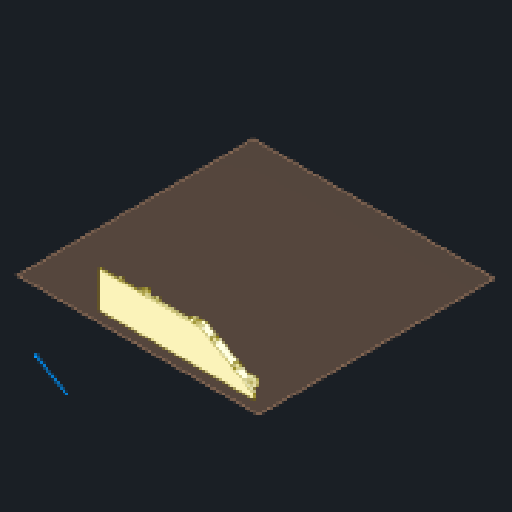
# Autodesk Inventor part: right_side
Saved by Autodesk Inventor 2023 (Build 270158000, 158)
## iProperties
Created: 2024-05-08
Part Number: right_side
Material: Nylon 6/6
Document SubType Name: Modeling
Designer: szymo
Density: 1.13 g/cm^3
Appearance: Nylon 6
Mass: 14.3001 g
Surface Area: 114.851 cm^2
Volume: 12.655 cm^3
Author: szymo
Autodesk Inventor part; units mm, degrees
ref_plane "YZ Plane" through (0, 0, 0) normal (1, 0, 0) x (0, 1, 0)
ref_plane "XZ Plane" through (0, 0, 0) normal (0, 1, 0) x (-1, 0, 0)
ref_plane "XY Plane" through (0, 0, 0) normal (0, 0, 1) x (1, 0, 0)
sketch "Sketch1" plane through (0, 0, 0) normal (0, 0, 1) x (1, 0, 0)
  line L0 (128, 8) -> (128, 3.5) projected
  line L1 (128, 3.5) -> (132, 3.5) projected
  line L2 (132, 3.5) -> (132, 0) projected
  line L3 (132, 0) -> (146, 0) projected
  line L4 (146, 0) -> (132, 9) projected
  line L5 (132, 9) -> (132, 8) projected
  line L6 (132, 8) -> (128, 8) projected
  circle A0 centre (-25, 12) radius 22.5 projected
  line L7 (116.5, 3.5) -> (116.5, 11.1395) projected
  line L8 (116.5, 14.6395) -> (116.5, 11.1395) projected
  line L9 (109.1155, 18.903) -> (116.5, 14.6395) projected
  line L10 (109.1155, 18.903) -> (83.8327, 33.5) projected
  line L11 (47.75, 33.5) -> (83.8327, 33.5) projected
  line L12 (0, 3.5) -> (0, 31) projected
  line L13 (0, 3.5) -> (0, 33.5)
  line L14 (0, 33.5) -> (83.8327, 33.5)
  line L15 (83.8327, 33.5) -> (128, 8)
  line L16 (128, 3.5) -> (0, 3.5)
  point P0 (0, 0)
  constraints: 8 end point, 2 collinear, 1 parallel, 1 point on line
extrude "Extrusion1" add sketch "Sketch1" against normal blind 2 contours L0 L16 L7 L8 L15 | L8 L7 L16 L12 L13 L14 L11 L10 L9
sketch "Sketch2" plane through (0, 0, -2) normal (0, 0, -1) x (-1, 0, 0)
  circle A0 centre (-15.375, 18.875) radius 13.7 projected
  line L0 (0, 33.5) -> (-83.8327, 33.5) projected
  line L1 (-128, 3.5) -> (0, 3.5) projected
  line L2 (-32.075, 33.5) -> (0, 33.5)
  line L3 (0, 33.5) -> (0, 3.5)
  line L4 (0, 3.5) -> (-32.075, 3.5)
  line L5 (-32.075, 3.5) -> (-32.075, 33.5)
  point P0 (0, 0)
  point P1 (-116.5, 3.5)
  dimension "d2" = 27.4
  dimension "d3" = 16.7
  constraints: 8 end point, 2 parallel, 1 horizontal, 1 perpendicular, 1 point on line
  measures "d2" diameter of A0
  measures "d3" distance from line of L5 A0.centre
extrude "Extrusion2" cut sketch "Sketch2" against normal blind 1 contours A0 | L3 L1 L5 L0
sketch "Sketch3" plane through (0, 0, -1) normal (0, 0, -1) x (-1, 0, 0)
  circle A0 centre (-15.375, 18.875) radius 13.7 projected
  line L0 (-32.075, 33.5) -> (0, 33.5) projected
  line L1 (-32.075, 3.5) -> (-32.075, 33.5) projected
  line L2 (0, 3.5) -> (-32.075, 3.5) projected
  line L3 (0, 33.5) -> (0, 3.5) projected
  line L4 (0, 3.5) -> (-128, 3.5) projected
  line L5 (0, 3.5) -> (-5, 3.5)
  line L6 (-5, 3.5) -> (-5, 6.5)
  line L7 (-5, 6.5) -> (0, 6.5)
  line L8 (0, 6.5) -> (0, 3.5)
  line L9 (-32.075, 3.5) -> (-27.075, 3.5)
  line L10 (-27.075, 3.5) -> (-27.075, 6.5)
  line L11 (-27.075, 6.5) -> (-32.075, 6.5)
  line L12 (-32.075, 6.5) -> (-32.075, 3.5)
  line L13 (-32.075, 9.5) -> (-25.365, 9.5)
  line L14 (-1.6801, 18.5) -> (0, 18.5)
  line L15 (0, 33.5) -> (0, 3.5) projected
  point P0 (0, 0)
  point P1 (-116.5, 3.5)
  point P2 (0, 18.5)
  dimension "d6" = 5
  dimension "d7" = 3
  dimension "d8" = 5
  dimension "d9" = 3
  dimension "d10" = 3
  constraints: 20 end point, 4 parallel, 3 perpendicular, 3 point on line, 2 horizontal, 2 point on circle, 1 midpoint
  measures "d6" distance of L6.end L7.end
  measures "d7" distance of L5.end L6.end
  measures "d8" distance of L11.end L10.end
  measures "d9" distance of L10.end L9.end
  measures "d10" distance between parallel lines of L13 L11
ref_plane "Work Plane1" through (1, 4.5, -18.6) normal (0, 0, 1) x (1, 0, 0)
ref_plane "Work Plane2" through (1.675, 5.175, -4.8) normal (0, 0, 1) x (1, 0, 0)
extrude "Extrusion3" add sketch "Sketch3" along normal blind 6.8 contours A0 L14 L3 L7 L6 L2 L10 L11 L1 L13 | L11 L10 L2 L1 | L3 L2 L6 L7
sketch "Sketch4" plane through (0, 0, -7.8) normal (0, 0, -1) x (-1, 0, 0)
  circle A0 centre (-15.375, 18.875) radius 13.7 projected
  line L0 (-1.6801, 18.5) -> (0, 18.5) projected
  line L1 (0, 33.5) -> (0, 18.5) projected
  line L2 (-32.075, 33.5) -> (0, 33.5) projected
  line L3 (-32.075, 9.5) -> (-32.075, 33.5) projected
  line L4 (-32.075, 9.5) -> (-25.365, 9.5) projected
  arc A1 (-25.365, 9.5) -> (-1.6801, 18.5) centre (-15.375, 18.875) ccw projected
  line L5 (-29.0741, 19.0336) -> (-32.075, 19.0336)
  line L6 (-32.075, 9.5) -> (-32.075, 33.5) projected
  line L7 (0, 18.5) -> (-1.6801, 18.5) projected
  line L8 (-1.6801, 18.5) -> (0, 18.5)
  arc A2 (-25.365, 9.5) -> (-1.6801, 18.5) centre (-15.375, 18.875) ccw projected
  line L9 (-25.365, 9.5) -> (-32.075, 9.5) projected
  line L10 (-32.075, 9.5) -> (-32.075, 3.5) projected
  line L11 (-32.075, 3.5) -> (0, 3.5) projected
  line L12 (0, 3.5) -> (0, 18.5) projected
  line L13 (0, 18.5) -> (-1.6801, 18.5) projected
  point P0 (0, 0)
  constraints: 4 end point, 1 collinear, 1 perpendicular, 1 point on line, 2 other
ref_plane "Work Plane3" through (1, 4.5, -18.6) normal (0, 0, 1) x (1, 0, 0)
extrude "Extrusion4" add sketch "Sketch4" along normal up to surface (10.8 mm away) contours A0 L4 L3 L5 | L0 L12 L11 L10 L4 A0
sketch "Sketch5" plane through (25.365, 9.5, -1) normal (0, 1, 0) x (1, 0, 0)
  line L0 (6.71, 0) -> (0, 0) projected
  line L1 (6.71, 1) -> (6.71, 0) projected
  line L2 (6.71, 1) -> (6.71, 6.8) projected
  line L3 (0, 6.8) -> (6.71, 6.8) projected
  line L4 (0, 0) -> (0, 6.8) projected
  line L5 (6.71, 0) -> (0, 6.8)
  line L6 (-0.1811, 0) -> (6.71, 6.8)
  point P0 (-25.365, -1)
  point P1 (3.2645, 3.4)
  constraints: 4 end point, 1 midpoint, 1 perpendicular, 1 point on line
hole "Hole1" at (28.6294, 9.5, -4.4) direction (0, -1, 0) diameter 3.6 end through all countersink diameter 6.5 countersink angle 90 clearance for "Countersunk Flat Head Screw ISO 2009/7046" size "M3" standard "ISO"
ref_plane "Work Plane4" through (41, 3.5, -89) normal (0, 1, 0) x (-1, 0, 0)
sketch "Sketch6" plane through (41, 3.5, -89) normal (0, 1, 0) x (-1, 0, 0)
  line L0 (8.925, 87) -> (-42.8327, 87) projected
  line L1 (-42.8327, 87) -> (-87, 87) projected
  line L2 (-87, 87) -> (8.925, 87) projected
  line L3 (-71, 89) -> (-71, 74) projected
  line L4 (-71, 74) -> (-87, 74) projected
  line L5 (-71, 87) -> (-64, 87)
  line L6 (-64, 87) -> (-64, 77)
  line L7 (-64, 77) -> (-71, 77)
  line L8 (-71, 77) -> (-71, 87)
  point P0 (41, 89)
  point P1 (-64, 87)
  dimension "d22" = 7
  dimension "d23" = 10
  constraints: 8 end point, 2 parallel, 2 point on line, 1 horizontal, 1 perpendicular
  measures "d22" distance of L6.end L7.end
  measures "d23" distance of L5.end L6.end
extrude "Extrusion5" add sketch "Sketch6" along normal blind 5
sketch "Sketch7" plane through (0, 0, -2) normal (0, 0, -1) x (-1, 0, 0)
  line L0 (-105, 8.5) -> (-105, 3.5) projected
  line L1 (-105, 3.5) -> (-32.075, 3.5) projected
  line L2 (-32.075, 3.5) -> (-32.075, 9.5) projected
  line L3 (-32.075, 9.5) -> (-32.075, 33.5) projected
  line L4 (-32.075, 33.5) -> (-83.8327, 33.5) projected
  line L5 (-83.8327, 33.5) -> (-128, 8) projected
  line L6 (-128, 8) -> (-128, 3.5) projected
  line L7 (-128, 3.5) -> (-112, 3.5) projected
  line L8 (-112, 3.5) -> (-112, 8.5) projected
  line L9 (-112, 8.5) -> (-105, 8.5) projected
  line L10 (-118.25, 3.5) -> (-115.75, 3.5) projected
  line L11 (-115.75, 3.5) -> (-118.25, 3.5)
  line L12 (-118.25, 3.5) -> (-118.25, 8.5)
  line L13 (-118.25, 8.5) -> (-115.75, 8.5)
  line L14 (-115.75, 8.5) -> (-115.75, 3.5)
  line L15 (-114, 3.5) -> (-120, 3.5)
  line L16 (-120, 3.5) -> (-120, 8.5)
  line L17 (-120, 8.5) -> (-114, 8.5)
  line L18 (-114, 8.5) -> (-114, 3.5)
  line L19 (-112, 8.5) -> (-114, 8.5)
  point P0 (0, 0)
  dimension "d26" = 5
  dimension "d27" = 6
  dimension "d28" = 1.75
  dimension "d29" = 1.75
  constraints: 18 end point, 4 parallel, 2 coincident, 2 horizontal, 2 perpendicular, 2 point on line, 1 collinear
  measures "d26" distance of L11.end L12.end
  measures "d27" distance of L16.end L17.end
  measures "d28" distance between parallel lines of L16 L12
  measures "d29" distance between parallel lines of L14 L18
extrude "Extrusion6" add sketch "Sketch7" along normal blind 10 contours L8 L7 L18 L19 | L18 L7 L14 L17 | L14 L7 L12 L13 | L12 L7 L16 L17
sketch "Sketch8" plane through (41, 8.5, -89) normal (0, 1, 0) x (1, 0, 0)
  line L0 (64, -77) -> (64, -87) projected
  line L1 (79, -87) -> (64, -87) projected
  line L2 (79, -87) -> (79, -77) projected
  line L3 (64, -77) -> (79, -77) projected
  line L4 (71, -77) -> (64, -83)
  line L5 (71, -89) -> (71, -74) projected
  point P0 (-41, -89)
  point P1 (67.5, -80)
  dimension "d40" = 4
  constraints: 3 point on line, 2 end point, 1 midpoint
  measures "d40" distance from line of L1 L4.end
hole "Hole2" at (108.5, 8.5, -9) direction (0, -1, 0) diameter 3.6 end through all countersink diameter 6 countersink angle 90 clearance for "Countersunk Flat Head Screw ISO 2009/7046" size "M3" standard "ISO"
sketch "Sketch9" plane through (0, 0, -2) normal (0, 0, -1) x (-1, 0, 0)
  line L0 (-120, 3.5) -> (-120, 8.5) projected
  line L1 (-120, 8.5) -> (-105, 8.5) projected
  line L2 (-105, 8.5) -> (-105, 3.5) projected
  line L3 (-105, 3.5) -> (-32.075, 3.5) projected
  line L4 (-32.075, 3.5) -> (-32.075, 9.5) projected
  line L5 (-32.075, 9.5) -> (-32.075, 33.5) projected
  line L6 (-32.075, 33.5) -> (-83.8327, 33.5) projected
  line L7 (-83.8327, 33.5) -> (-128, 8) projected
  line L8 (-128, 8) -> (-128, 3.5) projected
  line L9 (-128, 3.5) -> (-120, 3.5) projected
  line L10 (-73.8327, 33.5) -> (-125.7942, 3.5)
  line L11 (-105, 8.5) -> (-105, 15.5056)
  line L12 (0, 3.5) -> (-128, 3.5) projected
  line L13 (-128, 3.5) -> (-120, 3.5)
  line L14 (-120, 6.8453) -> (-120, 3.5)
  line L15 (-120, 6.8453) -> (-120, 8.5)
  line L16 (-120, 8.5) -> (-105, 8.5)
  line L17 (-122, 3.5) -> (-122, 11.4641)
  line L18 (-122, 3.5) -> (-114.0359, 3.5) construction
  line L19 (-32.075, 33.5) -> (0, 33.5) projected
  line L20 (-120, 8.5) -> (-120, 12.6188)
  line L21 (-73.8327, 33.5) -> (-32.075, 5.3098)
  line L22 (-75.2777, 32.6657) -> (-32.075, 3.5) construction
  line L23 (-76.7228, 31.8314) -> (-34.7559, 3.5)
  line L24 (-76.7228, 31.8314) -> (-76.7228, 3.5) construction
  line L25 (-78.2228, 30.9654) -> (-78.2228, 3.5)
  line L26 (-75.2228, 30.8188) -> (-75.2228, 3.5)
  line L27 (-78.2228, 3.5) -> (-99.1114, 18.9053) construction
  line L28 (-97.6939, 19.7237) -> (-78.2228, 5.3638)
  line L29 (-100.5289, 18.0869) -> (-80.75, 3.5)
  line L30 (-75.2228, 30.8188) -> (-54.9893, 3.5) construction
  line L31 (-75.2228, 28.2985) -> (-56.8559, 3.5)
  line L32 (-71.4895, 28.2985) -> (-53.1227, 3.5)
  line L33 (-105, 5.5) -> (-32.075, 5.5)
  line L34 (-32.075, 9.5) -> (-36.1077, 8.0322)
  line L35 (-39.5912, 6.7643) -> (-43.0649, 5.5)
  point P0 (0, 0)
  point P1 (-128, 5.75)
  point P2 (-75.2228, 3.5)
  point P3 (-34.7559, 3.5)
  point P4 (-53.1227, 3.5)
  point P5 (-56.8559, 3.5)
  point P6 (-37.7184, 5.5)
  point P7 (-54.604, 5.5)
  point P8 (-58.3372, 5.5)
  point P9 (-75.2228, 5.5)
  point P10 (-83.4618, 5.5)
  point P11 (-32.3567, 5.5)
  dimension "d39" = 5
  dimension "d41" = 90
  dimension "d42" = 6
  dimension "d51" = 1.5
  dimension "d52" = 1.5
  dimension "d53" = 1.5
  dimension "d54" = 1.5
  dimension "d55" = 22.1042
  dimension "d56" = 22.1042
  dimension "d57" = 1.5
  dimension "d58" = 1.5
  dimension "d59" = 20.2335
  dimension "d60" = 20.2335
  dimension "d61" = 1.5
  dimension "d62" = 1.5
  dimension "d96" = 2
  dimension "d97" = 70
  constraints: 46 end point, 16 point on line, 6 parallel, 5 collinear, 5 perpendicular, 2 vertical, 1 horizontal, 1 midpoint, 21 other
  measures "d41" angle of L18 L17
  measures "d42" distance from line of L17 point (-128, 5.75)
  measures "d51" distance between parallel lines of L22 L21
  measures "d52" distance between parallel lines of L22 L23
  measures "d53" distance between parallel lines of L24 L26
  measures "d54" distance between parallel lines of L24 L25
  measures "d55" distance from line of L27 L25.start
  measures "d56" distance from line of L14.start L27
  measures "d57" distance between parallel lines of L27 L28
  measures "d58" distance between parallel lines of L27 L29
  measures "d59" distance of L26.end L30.end
  measures "d60" distance of L30.end L23.end
  measures "d61" distance between parallel lines of L30 L32
  measures "d62" distance between parallel lines of L30 L31
  measures "d97" angle of L34 L4
extrude "zeberka" add sketch "Sketch9" along normal blind 4 contours L2 L33 L29 L3 | L20 L7 L6 L10 L1 | L10 L11 L1 | L29 L33 L28 L25 L3 | L29 L10 L28 L33 | L25 L33 L26 L3 | L26 L33 L31 L3 | L21 L33 L23 L10 | L25 L10 L23 L26 L33 | L31 L33 L32 L3 | L34 L4 L33 L21 | L32 L33 L23 L3 | L31 L26 L23 L32 L33 | L21 L4 L3 L23 L33 | L33 L35 L23
sketch "Sketch11" plane through (0, 0, -2) normal (0, 0, -1) x (-1, 0, 0)
  line L0 (-32.075, 9.5) -> (-32.075, 33.5) projected
  line L1 (-32.075, 33.5) -> (-38.075, 33.5)
  line L2 (-38.075, 33.5) -> (-38.075, 27.5)
  line L3 (-38.075, 27.5) -> (-32.075, 27.5)
  line L4 (-32.075, 27.5) -> (-32.075, 33.5)
  point P0 (0, 0)
  dimension "d63" = 6
  dimension "d64" = 6
  constraints: 8 end point, 2 parallel, 1 horizontal, 1 perpendicular
  measures "d63" distance of L3.end L2.end
  measures "d64" distance of L2.end L1.end
extrude "Extrusion8" add sketch "Sketch11" along normal blind 4
fillet "Fillet1" radius 3 3 edges at (38.075, 30.5, -2) (38.075, 30.5, -6) (32.075, 30.5, -6)
chamfer "Chamfer1" distance 4 angle 45 2 edges at (39.575, 27.5, -2) (35.075, 27.5, -2)
sketch "Sketch13" plane through (0, 33.5, 0) normal (0, 1, 0) x (1, 0, 0)
  arc A0 (38.2466, 4) -> (35.4181, 6) centre (35.4181, 3) ccw projected
  line L0 (35.075, 6) -> (35.4181, 6) projected
  arc A1 (35.075, 6) -> (32.075, 3) centre (35.075, 3) ccw projected
  line L1 (32.075, 3) -> (32.075, 1) projected
  line L2 (32.075, 1) -> (0, 1) projected
  line L3 (0, 0) -> (0, 1) projected
  line L4 (83.8327, 0) -> (0, 0) projected
  line L5 (83.8327, 0) -> (83.8327, 6) projected
  line L6 (73.8327, 6) -> (83.8327, 6) projected
  line L7 (73.8327, 2) -> (73.8327, 6) projected
  line L8 (41.075, 2) -> (73.8327, 2) projected
  arc A2 (38.2466, 4) -> (41.075, 2) centre (41.075, 5) ccw projected
  line L9 (73.8327, 2) -> (73.8327, 0)
  line L10 (0, 0) -> (128, 0) projected
  constraints: 2 end point, 1 perpendicular, 1 point on line
extrude "Extrusion9" add sketch "Sketch13" against normal blind 5.75 contours L7 L6 L5 L4 L9
sketch "Sketch14" plane through (0, 33.5, 0) normal (0, 1, 0) x (1, 0, 0)
  line L0 (41.075, 2) -> (73.8327, 2) projected
  arc A0 (38.2466, 4) -> (41.075, 2) centre (41.075, 5) ccw projected
  arc A1 (38.2466, 4) -> (35.4181, 6) centre (35.4181, 3) ccw projected
  line L1 (35.075, 6) -> (35.4181, 6) projected
  arc A2 (35.075, 6) -> (32.075, 3) centre (35.075, 3) ccw projected
  line L2 (32.075, 3) -> (32.075, 1) projected
  line L3 (32.075, 1) -> (0, 1) projected
  line L4 (0, 0) -> (0, 1) projected
  line L5 (83.8327, 0) -> (0, 0) projected
  line L6 (83.8327, 0) -> (83.8327, 6) projected
  line L7 (73.8327, 6) -> (83.8327, 6) projected
  line L8 (73.8327, 2) -> (73.8327, 6) projected
  line L9 (73.8327, 6) -> (83.8327, 0)
  point P0 (0, 0)
  point P1 (35.2466, 3)
  point P2 (78.8327, 3)
  constraints: 2 end point, 1 midpoint
hole "Hole4" at (35.2466, 33.5, -3) at (78.8327, 33.5, -3) direction (0, -1, 0) diameter 4 depth 5 counterbore diameter 4.6 counterbore depth 1
sketch "Sketch15" plane through (128, 8, 0) normal (0.5, 0.8660254, 0) x (0.8660254, -0.5, 0)
  line L0 (0, 0) -> (-51, 0) projected
  line L1 (0, 0) -> (0, 2) projected
  line L2 (-9.2376, 2) -> (0, 2) projected
  line L3 (-9.2376, 2) -> (-9.2376, 6) projected
  line L4 (-51, 6) -> (-9.2376, 6) projected
  line L5 (-51, 0) -> (-51, 6) projected
  line L6 (-108.6013, 0) -> (2.25, 0) projected
  line L7 (-30.1188, 0) -> (-30.1188, 6)
  line L8 (-9.2376, 6) -> (-9.2376, 0)
  line L9 (-51, 6) -> (-30.1188, 0)
  line L10 (-30.1188, 6) -> (-51, 0)
  line L11 (-30.1188, 0) -> (-9.2376, 6)
  line L12 (-30.1188, 6) -> (-9.2376, 0)
  point P0 (-106.8513, 0)
  point P1 (-19.6782, 3)
  point P2 (-40.5594, 3)
  dimension "d87" = 20.8812
  dimension "d88" = 20.8812
  constraints: 12 end point, 3 midpoint, 2 parallel, 2 perpendicular, 2 point on line
  measures "d87" distance between parallel lines of L5 L7
  measures "d88" distance between parallel lines of L8 L7
hole "Hole5" at (110.9582, 17.8391, -3) at (92.8745, 28.2797, -3) direction (-0.5, -0.8660254, 0) diameter 4 depth 4.75 counterbore diameter 4.6 counterbore depth 0.75
equation "\"d28\" = d29"
equation "\"d52\" = d51"
equation "\"d54\" = d53"
equation "\"d58\" = d57"
equation "\"d62\" = d61"
equation "\"d87\" = d88"
body "Solid1"
